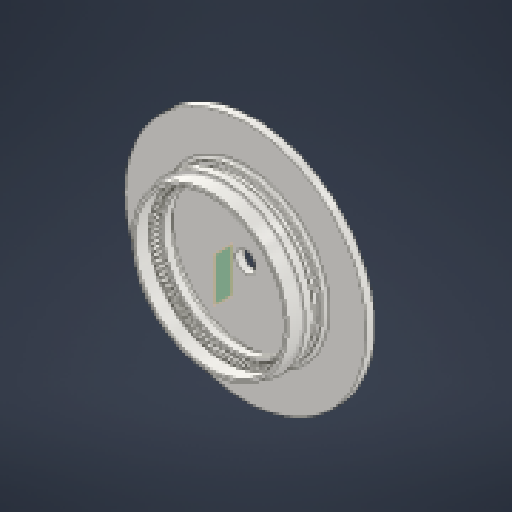
# Autodesk Inventor part: 스퍼 기어1
Saved by Autodesk Inventor 2026.1 (Build 301233020, 233B)
## iProperties
CustomPartVersion: 1
Created: 2025-11-12
Part Number: 스퍼 기어1
Material: Steel
Document SubType Name: Modeling
Designer: jaewook
Categories: <?xml version="1.0" encoding="UTF-16"?> <MemberInstance><Categories><FamilyTemplate><FamilyTemplateParameter ValueType="xs:double" Id="1" ObjectReferenceKey="da_z" ObjectType="kUserParameterObject"/><FamilyTemplateParameter ValueType="xs:double" Id="2" ObjectReferenceKey="da_b" ObjectType="kUserParameterObject"/><FamilyTemplateParameter ValueType="xs:double" Id="3" ObjectReferenceKey="da_beta" ObjectType="kUserParameterObject"/><FamilyTemplateParameter ValueType="xs:double" Id="4" ObjectReferenceKey="da_da" ObjectType="kUserParameterObject"/><FamilyTemplateParameter ValueType="xs:double" Id="5" ObjectReferenceKey="da_aw" ObjectType="kUserParameterObject"/><FamilyTemplateParameter ValueType="xs:string" Id="6" ObjectReferenceKey="EAIAABAAAACIAQAAAAAAAIAAAAAAAAAA" ObjectType="83910656" SubObjectId="SurfaceGeometry"/></FamilyTemplate><ParamToTemplateMap><ParamToTemplate CategoryParameter="//CategoryParameter[@InternalName='046C89C9-8512-4d59-83FE-43B91F4F132A']" TemplateParameter="1"/><ParamToTemplate CategoryParameter="//CategoryParameter[@InternalName='2552DF32-E462-4b46-AEBF-C6C7768E72AC']" TemplateParameter="2"/><ParamToTemplate CategoryParameter="//CategoryParameter[@InternalName='C9EE641D-15FC-4fae-A226-E94C4372FDD7']" TemplateParameter="3"/><ParamToTemplate><ParamToTemplate CategoryParameter="//CategoryParameter[@InternalName='00B6519A-459B-49c7-AD84-2E56D39A5744']" ConstantValue="0.000000"/></ParamToTemplate><ParamToTemplate><ParamToTemplate CategoryParameter="//CategoryParameter[@InternalName='04B31F0E-C7A6-4894-AA32-9629BEFACF47']" ConstantValue="0.950000"/></ParamToTemplate><ParamToTemplate><ParamToTemplate CategoryParameter="//CategoryParameter[@InternalName='43CBEC2E-7847-49e7-A936-2F7889FCB2D9']" ConstantValue="0.250000"/></ParamToTemplate><ParamToTemplate><ParamToTemplate CategoryParameter="//CategoryParameter[@InternalName='B1EFC894-105D-4ebd-86BF-FA20ED196853']" ConstantValue="0.379900"/></ParamToTemplate><ParamToTemplate><ParamToTemplate CategoryParameter="//CategoryParameter[@InternalName='51175063-3D10-4879-93E8-6246FE8B403D']" ConstantValue="2060000000.000000"/></ParamToTemplate><ParamToTemplate><ParamToTemplate CategoryParameter="//CategoryParameter[@InternalName='A3A52E27-4454-46a9-B0BD-C932399B70AF']" ConstantValue="0.300000"/></ParamToTemplate><ParamToTemplate><ParamToTemplate CategoryParameter="//CategoryParameter[@InternalName='91B76062-C214-41d9-B1B9-14D2AB99603D']" ConstantValue="0.200000"/></ParamToTemplate><ParamToTemplate><ParamToTemplate CategoryParameter="//CategoryParameter[@InternalName='374E806E-8B8A-4dda-A9AA-1039D6500AD2']" ConstantValue="5.000000"/></ParamToTemplate><ParamToTemplate><ParamToTemplate CategoryParameter="//CategoryParameter[@InternalName='2D373A89-B862-43d6-8D0B-0CBF12AB9F6C']" ConstantValue="0.349066"/></ParamToTemplate><ParamToTemplate CategoryParameter="//CategoryParameter[@InternalName='37777632-D6A2-4fac-9D53-DB8ACD95C989']" TemplateParameter="4"/><ParamToTemplate CategoryParameter="//CategoryParameter[@InternalName='FD1017F1-B727-4f7e-9707-0F86F1FF9423']" TemplateParameter="5"/><ParamToTemplate><ParamToTemplate CategoryParameter="//CategoryParameter[@InternalName='9E1B4470-B2D3-4ff1-B813-535BB4CDF51A']" ConstantValue="3520000.000000"/></ParamToTemplate><ParamToTemplate><ParamToTemplate CategoryParameter="//CategoryParameter[@InternalName='F8452263-BFF6-458c-9FB1-07C4B99E95CD']" ConstantValue="11400000.000000"/></ParamToTemplate><ParamToTemplate><ParamToTemplate CategoryParameter="//CategoryParameter[@InternalName='3E3BB259-FD49-497f-8171-6EBC954A3479']" ConstantValue="2.000000"/></ParamToTemplate><ParamToTemplate CategoryParameter="//CategoryParameter[@InternalName='27C3BAF2-7550-4e4b-AE2C-0DB134B7D9B7']" TemplateParameter="6"/></ParamToTemplateMap><Category DisplayName="Gear" InternalName="DC85795E-93AB-48d5-8EEE-5A27447B64BD" Mnemonic="Gear"><CategoryParameter DisplayName="z" InternalName="046C89C9-8512-4d59-83FE-43B91F4F132A" Mnemonic="z"/><CategoryParameter DisplayName="b" InternalName="2552DF32-E462-4b46-AEBF-C6C7768E72AC" Mnemonic="b"/><CategoryParameter DisplayName="||b|" InternalName="C9EE641D-15FC-4fae-A226-E94C4372FDD7" Mnemonic="beta"/><CategoryParameter DisplayName="x" InternalName="00B6519A-459B-49c7-AD84-2E56D39A5744" Mnemonic="x"/><CategoryParameter DisplayName="a*" InternalName="04B31F0E-C7A6-4894-AA32-9629BEFACF47" Mnemonic="a"/><CategoryParameter DisplayName="c*" InternalName="43CBEC2E-7847-49e7-A936-2F7889FCB2D9" Mnemonic="c"/><CategoryParameter DisplayName="r|.f|*" InternalName="B1EFC894-105D-4ebd-86BF-FA20ED196853" Mnemonic="rf"/><CategoryParameter DisplayName="E" InternalName="51175063-3D10-4879-93E8-6246FE8B403D" Mnemonic="E"/><CategoryParameter DisplayName="||m|" InternalName="A3A52E27-4454-46a9-B0BD-C932399B70AF" Mnemonic="mi"/><Category DisplayName="SpurGear" InternalName="26C5A22E-A91E-4dfd-A3B3-23CCAFAE1764" Mnemonic="SpurGear"><CategoryParameter DisplayName="m" InternalName="91B76062-C214-41d9-B1B9-14D2AB99603D" Mnemonic="m"/><CategoryParameter DisplayName="P" InternalName="374E806E-8B8A-4dda-A9AA-1039D6500AD2" Mnemonic="PP"/><CategoryParameter DisplayName="||a|" InternalName="2D373A89-B862-43d6-8D0B-0CBF12AB9F6C" Mnemonic="alpha"/><CategoryParameter DisplayName="d|.a|" InternalName="37777632-D6A2-4fac-9D53-DB8ACD95C989" Mnemonic="da"/><CategoryParameter DisplayName="a|.w|" InternalName="FD1017F1-B727-4f7e-9707-0F86F1FF9423" Mnemonic="aw"/><CategoryParameter DisplayName="||s||.Flim|" InternalName="9E1B4470-B2D3-4ff1-B813-535BB4CDF51A" Mnemonic="sFlim"/><CategoryParameter DisplayName="||s||.Hlim|" InternalName="F8452263-BFF6-458c-9FB1-07C4B99E95CD" Mnemonic="sHlim"/><CategoryParameter DisplayName="유형" InternalName="3E3BB259-FD49-497f-8171-6EBC954A3479" Mnemonic="type"/><Category DisplayName="InternalSpurGear" InternalName="7CF704F6-14A9-42f8-93CE-E71DF57C2B55" Mnemonic="InternalSpurGear"><CategoryParameter DisplayName="PitchDiameter" InternalName="27C3BAF2-7550-4e4b-AE2C-0DB134B7D9B7" Mnemonic="IDS_PITCHDIAM"/></Category></Category></Category></Categories></MemberInstance>
Density: 1 g/cm^3
Appearance: Steel
d16: 70.000 mm
d17: 0.000 mm
d45: 0.000 mm
d47: 70.000 mm
d50: 0.000 mm
d51: 0.000 mm
d52: 70.000 mm
Author: jaewook
Autodesk Inventor part; units mm, degrees
sketch "Sketch1" plane through (0, 0, 0) normal (0, 0, 1) x (1, 0, 0)
  circle A0 centre (0, 0) radius 97.02
  dimension "d0" = 194.04
  constraints: 1 centre point
  measures "d0" diameter of A0
extrude "Extrusion1" add sketch "Sketch1" along normal blind 10
ref_plane "Work Plane2" through (0, 0, 5) normal (0, 0, 1) x (1, 0, 0)
sketch "Sketch2" plane through (0, 0, 0) normal (0, 0, -1) x (-1, 0, 0)
  circle A0 centre (0, 0) radius 97.02 projected
  circle A1 centre (0, 0) radius 90
  dimension "d3" = 180
  constraints: 1 centre point, 1 coincident
  measures "d3" diameter of A1
surface extrude "피치 지름" sketch "Sketch2" against normal through all shown no curves A1
ref_plane "Work Plane8" through (0, 0, 0) normal (0.9993908, 0.0348995, 0) x (0, 0, 1)
ref_plane "Work Plane9" through (0, 0, 0) normal (1, 0, 0) x (0, 1, 0)
spur gear teeth "스퍼 기어" teeth 90 pitch diameter 180 tip diameter 176.2 root diameter 184.8 face width 10 start plane through (0, 0, 0) normal (0, 0, -1) x (-1, 0, 0)
sketch "스케치14" plane through (0, 0, 10) normal (0, 0, 1) x (1, 0, 0)
  circle A0 centre (0, 0) radius 97.02 projected
  circle A1 centre (0, 0) radius 93.02
  dimension "d81" = 4
  constraints: 1 centre point, 1 coincident
  measures "d81" radial gap between concentric circles of A1 A0
extrude "돌출9" add sketch "스케치14" along normal blind 17
sketch "스케치15" plane through (0, 0, 0) normal (0, 0, -1) x (-1, 0, 0)
  circle A0 centre (0, 0) radius 97.02 projected
  circle A1 centre (0, 0) radius 92.4
  circle A2 centre (0, 0) radius 95.02
  circle A3 centre (0, 0) radius 85
  dimension "d84" = 184.8
  dimension "d85" = 190.04
  dimension "d86" = 170
  constraints: 3 centre point, 3 coincident
  measures "d84" diameter of A1
  measures "d85" diameter of A2
  measures "d86" diameter of A3
extrude "돌출10" add sketch "스케치15" along normal blind 10 contours A1 | A2
sketch "스케치16" plane through (0, 0, -10) normal (0, 0, -1) x (-1, 0, 0)
  circle A0 centre (0, 0) radius 95.02 projected
  circle A1 centre (0, 0) radius 85 projected
  circle A2 centre (0, 0) radius 90.78
  dimension "d89" = 4.24
  constraints: 1 centre point, 1 coincident
  measures "d89" radial gap between concentric circles of A2 A0
extrude "돌출11" add sketch "스케치16" along normal blind 1 contours A0
sketch "스케치17" plane through (0, 0, -11) normal (0, 0, -1) x (-1, 0, 0)
  circle A0 centre (0, 0) radius 90.78 projected
  circle A1 centre (0, 0) radius 85 projected
  circle A2 centre (0, 0) radius 100.02
  circle A3 centre (0, 0) radius 95.02 projected
  dimension "d150" = 5
  constraints: 1 centre point, 1 coincident
  measures "d150" radial gap between concentric circles of A2 A3
extrude "돌출12" add sketch "스케치17" along normal blind 6.5 contours A2 | A3
sketch "스케치18" plane through (0, 0, -17.5) normal (0, 0, -1) x (-1, 0, 0)
  circle A0 centre (0, 0) radius 90.78 projected
  circle A1 centre (0, 0) radius 150
  circle A2 centre (0, 0) radius 12.5
  dimension "d94" = 300
  dimension "d95" = 25
  constraints: 2 centre point, 2 coincident
  measures "d94" diameter of A1
  measures "d95" diameter of A2
extrude "돌출13" add sketch "스케치18" along normal blind 10 contours A0 | A1
fillet "모깎기2" radius 4 1 edges at (100.02, 0, -17.5)
sketch "스케치4" plane through (0, 0, 0) normal (0, 0, -1) x (-1, 0, 0)
  arc A0 (-13.6576, -91.3851) -> (-12.0606, -91.6095) centre (0, 0) ccw projected
  arc A1 (-19.999, -90.2098) -> (-18.4216, -90.545) centre (0, 0) ccw projected
  arc A2 (-26.243, -88.5949) -> (-24.6928, -89.0395) centre (0, 0) ccw projected
  arc A3 (-32.3592, -86.5485) -> (-30.8438, -87.1001) centre (0, 0) ccw projected
  arc A4 (-38.3177, -84.0804) -> (-36.8444, -84.7364) centre (0, 0) ccw projected
  arc A5 (-44.0895, -81.2027) -> (-42.6656, -81.9598) centre (0, 0) ccw projected
  arc A6 (-49.6465, -77.9294) -> (-48.2789, -78.784) centre (0, 0) ccw projected
  arc A7 (-54.9616, -74.2764) -> (-53.657, -75.2243) centre (0, 0) ccw projected
  arc A8 (-60.009, -70.2615) -> (-58.7736, -71.2981) centre (0, 0) ccw projected
  arc A9 (-64.764, -65.9043) -> (-63.604, -67.0246) centre (0, 0) ccw projected
  arc A10 (-69.2035, -61.2261) -> (-68.1244, -62.4245) centre (0, 0) ccw projected
  arc A11 (-73.3058, -56.2496) -> (-72.313, -57.5204) centre (0, 0) ccw projected
  arc A12 (-77.051, -50.999) -> (-76.1493, -52.3359) centre (0, 0) ccw projected
  arc A13 (-80.4209, -45.4999) -> (-79.6145, -46.8965) centre (0, 0) ccw projected
  arc A14 (-83.3989, -39.7792) -> (-82.6919, -41.2287) centre (0, 0) ccw projected
  arc A15 (-85.9706, -33.8647) -> (-85.3665, -35.3599) centre (0, 0) ccw projected
  arc A16 (-88.1234, -27.7852) -> (-87.6251, -29.319) centre (0, 0) ccw projected
  arc A17 (-89.847, -21.5704) -> (-89.4568, -23.1351) centre (0, 0) ccw projected
  arc A18 (-91.1328, -15.2504) -> (-90.8528, -16.8386) centre (0, 0) ccw projected
  arc A19 (-91.9746, -8.8561) -> (-91.806, -10.46) centre (0, 0) ccw projected
  arc A20 (-92.3683, -2.4188) -> (-92.3121, -4.0304) centre (0, 0) ccw projected
  arc A21 (-92.3121, 4.0304) -> (-92.3683, 2.4188) centre (0, 0) ccw projected
  arc A22 (-91.806, 10.46) -> (-91.9746, 8.8561) centre (0, 0) ccw projected
  arc A23 (-90.8528, 16.8386) -> (-91.1328, 15.2504) centre (0, 0) ccw projected
  arc A24 (-89.4568, 23.1351) -> (-89.847, 21.5704) centre (0, 0) ccw projected
  arc A25 (-87.6251, 29.319) -> (-88.1234, 27.7852) centre (0, 0) ccw projected
  arc A26 (-85.3665, 35.3599) -> (-85.9706, 33.8647) centre (0, 0) ccw projected
  arc A27 (-82.6919, 41.2287) -> (-83.3989, 39.7792) centre (0, 0) ccw projected
  arc A28 (-79.6145, 46.8965) -> (-80.4209, 45.4999) centre (0, 0) ccw projected
  arc A29 (-76.1493, 52.3359) -> (-77.051, 50.999) centre (0, 0) ccw projected
  arc A30 (-72.313, 57.5204) -> (-73.3058, 56.2496) centre (0, 0) ccw projected
  arc A31 (-68.1244, 62.4245) -> (-69.2035, 61.2261) centre (0, 0) ccw projected
  arc A32 (-63.604, 67.0246) -> (-64.764, 65.9043) centre (0, 0) ccw projected
  arc A33 (-58.7736, 71.2981) -> (-60.009, 70.2615) centre (0, 0) ccw projected
  arc A34 (-53.657, 75.2243) -> (-54.9616, 74.2764) centre (0, 0) ccw projected
  arc A35 (-48.2789, 78.784) -> (-49.6465, 77.9294) centre (0, 0) ccw projected
  arc A36 (-42.6656, 81.9598) -> (-44.0895, 81.2027) centre (0, 0) ccw projected
  arc A37 (-36.8444, 84.7364) -> (-38.3177, 84.0804) centre (0, 0) ccw projected
  arc A38 (-30.8438, 87.1001) -> (-32.3592, 86.5485) centre (0, 0) ccw projected
  arc A39 (-24.6928, 89.0395) -> (-26.243, 88.5949) centre (0, 0) ccw projected
  arc A40 (-18.4216, 90.545) -> (-19.999, 90.2098) centre (0, 0) ccw projected
  arc A41 (-12.0606, 91.6095) -> (-13.6576, 91.3851) centre (0, 0) ccw projected
  arc A42 (-5.6409, 92.2277) -> (-7.2496, 92.1152) centre (0, 0) ccw projected
  arc A43 (0.8063, 92.3965) -> (-0.8063, 92.3965) centre (0, 0) ccw projected
  arc A44 (7.2496, 92.1152) -> (5.6409, 92.2277) centre (0, 0) ccw projected
  arc A45 (13.6576, 91.3851) -> (12.0606, 91.6095) centre (0, 0) ccw projected
  arc A46 (19.999, 90.2098) -> (18.4216, 90.545) centre (0, 0) ccw projected
  arc A47 (26.243, 88.5949) -> (24.6928, 89.0395) centre (0, 0) ccw projected
  arc A48 (32.3592, 86.5485) -> (30.8438, 87.1001) centre (0, 0) ccw projected
  arc A49 (38.3177, 84.0804) -> (36.8444, 84.7364) centre (0, 0) ccw projected
  arc A50 (44.0895, 81.2027) -> (42.6656, 81.9598) centre (0, 0) ccw projected
  arc A51 (49.6465, 77.9294) -> (48.2789, 78.784) centre (0, 0) ccw projected
  arc A52 (54.9616, 74.2764) -> (53.657, 75.2243) centre (0, 0) ccw projected
  arc A53 (60.009, 70.2615) -> (58.7736, 71.2981) centre (0, 0) ccw projected
  arc A54 (64.764, 65.9043) -> (63.604, 67.0246) centre (0, 0) ccw projected
  arc A55 (69.2035, 61.2261) -> (68.1244, 62.4245) centre (0, 0) ccw projected
  arc A56 (73.3058, 56.2496) -> (72.313, 57.5204) centre (0, 0) ccw projected
  arc A57 (77.051, 50.999) -> (76.1493, 52.3359) centre (0, 0) ccw projected
  arc A58 (80.4209, 45.4999) -> (79.6145, 46.8965) centre (0, 0) ccw projected
  arc A59 (83.3989, 39.7792) -> (82.6919, 41.2287) centre (0, 0) ccw projected
  arc A60 (85.9706, 33.8647) -> (85.3665, 35.3599) centre (0, 0) ccw projected
  arc A61 (88.1234, 27.7852) -> (87.6251, 29.319) centre (0, 0) ccw projected
  arc A62 (89.847, 21.5704) -> (89.4568, 23.1351) centre (0, 0) ccw projected
  arc A63 (91.1328, 15.2504) -> (90.8528, 16.8386) centre (0, 0) ccw projected
  arc A64 (91.9746, 8.8561) -> (91.806, 10.46) centre (0, 0) ccw projected
  arc A65 (92.3683, 2.4188) -> (92.3121, 4.0304) centre (0, 0) ccw projected
  arc A66 (92.3121, -4.0304) -> (92.3683, -2.4188) centre (0, 0) ccw projected
  arc A67 (91.806, -10.46) -> (91.9746, -8.8561) centre (0, 0) ccw projected
  arc A68 (90.8528, -16.8386) -> (91.1328, -15.2504) centre (0, 0) ccw projected
  arc A69 (89.4568, -23.1351) -> (89.847, -21.5704) centre (0, 0) ccw projected
  arc A70 (87.6251, -29.319) -> (88.1234, -27.7852) centre (0, 0) ccw projected
  arc A71 (85.3665, -35.3599) -> (85.9706, -33.8647) centre (0, 0) ccw projected
  arc A72 (82.6919, -41.2287) -> (83.3989, -39.7792) centre (0, 0) ccw projected
  arc A73 (79.6145, -46.8965) -> (80.4209, -45.4999) centre (0, 0) ccw projected
  arc A74 (76.1493, -52.3359) -> (77.051, -50.999) centre (0, 0) ccw projected
  arc A75 (72.313, -57.5204) -> (73.3058, -56.2496) centre (0, 0) ccw projected
  arc A76 (68.1244, -62.4245) -> (69.2035, -61.2261) centre (0, 0) ccw projected
  arc A77 (63.604, -67.0246) -> (64.764, -65.9043) centre (0, 0) ccw projected
  arc A78 (58.7736, -71.2981) -> (60.009, -70.2615) centre (0, 0) ccw projected
  arc A79 (53.657, -75.2243) -> (54.9616, -74.2764) centre (0, 0) ccw projected
  arc A80 (48.2789, -78.784) -> (49.6465, -77.9294) centre (0, 0) ccw projected
  arc A81 (42.6656, -81.9598) -> (44.0895, -81.2027) centre (0, 0) ccw projected
  arc A82 (36.8444, -84.7364) -> (38.3177, -84.0804) centre (0, 0) ccw projected
  arc A83 (30.8438, -87.1001) -> (32.3592, -86.5485) centre (0, 0) ccw projected
  arc A84 (24.6928, -89.0395) -> (26.243, -88.5949) centre (0, 0) ccw projected
  arc A85 (18.4216, -90.545) -> (19.999, -90.2098) centre (0, 0) ccw projected
  arc A86 (12.0606, -91.6095) -> (13.6576, -91.3851) centre (0, 0) ccw projected
  arc A87 (5.6409, -92.2277) -> (7.2496, -92.1152) centre (0, 0) ccw projected
  arc A88 (-0.8063, -92.3965) -> (0.8063, -92.3965) centre (0, 0) ccw projected
  arc A89 (-7.2496, -92.1152) -> (-5.6409, -92.2277) centre (0, 0) ccw projected
  circle A90 centre (0, 0) radius 97.02 projected
  circle A91 centre (0, 0) radius 92.4
  point P0 (-92.3683, 2.4188)
  point P1 (-92.3121, 4.0304)
  point P2 (-91.9746, 8.8561)
  point P3 (-91.1328, 15.2504)
  point P4 (-89.847, 21.5704)
  point P5 (-88.1234, 27.7852)
  point P6 (-83.3989, 39.7792)
  point P7 (-80.4209, 45.4999)
  point P8 (-79.6145, 46.8965)
  point P9 (-76.1493, 52.3359)
  point P10 (-72.313, 57.5204)
  point P11 (-60.009, 70.2615)
  point P12 (-58.7736, 71.2981)
  point P13 (-54.9616, 74.2764)
  point P14 (-53.657, 75.2243)
  point P15 (-44.0895, 81.2027)
  point P16 (-38.3177, 84.0804)
  point P17 (-32.3592, 86.5485)
  point P18 (-26.243, 88.5949)
  point P19 (-24.6928, 89.0395)
  point P20 (-19.999, 90.2098)
  point P21 (-18.4216, 90.545)
  point P22 (-13.6576, 91.3851)
  point P23 (-12.0606, 91.6095)
  point P24 (-7.2496, 92.1152)
  point P25 (-0.8063, 92.3965)
  point P26 (0.8063, 92.3965)
  point P27 (5.6409, 92.2277)
  point P28 (7.2496, 92.1152)
  point P29 (12.0606, 91.6095)
  point P30 (18.4216, 90.545)
  point P31 (24.6928, 89.0395)
  point P32 (30.8438, 87.1001)
  point P33 (36.8444, 84.7364)
  point P34 (38.3177, 84.0804)
  point P35 (42.6656, 81.9598)
  point P36 (48.2789, 78.784)
  point P37 (49.6465, 77.9294)
  point P38 (54.9616, 74.2764)
  point P39 (58.7736, 71.2981)
  point P40 (63.604, 67.0246)
  point P41 (68.1244, 62.4245)
  point P42 (72.313, 57.5204)
  point P43 (73.3058, 56.2496)
  point P44 (79.6145, 46.8965)
  point P45 (80.4209, 45.4999)
  point P46 (85.3665, 35.3599)
  point P47 (87.6251, 29.319)
  point P48 (89.4568, 23.1351)
  point P49 (89.847, 21.5704)
  point P50 (90.8528, 16.8386)
  point P51 (91.1328, 15.2504)
  point P52 (91.806, 10.46)
  point P53 (91.9746, 8.8561)
  point P54 (92.3683, -2.4188)
  point P55 (92.3121, -4.0304)
  point P56 (91.9746, -8.8561)
  point P57 (91.1328, -15.2504)
  point P58 (89.847, -21.5704)
  point P59 (88.1234, -27.7852)
  point P60 (85.9706, -33.8647)
  point P61 (72.313, -57.5204)
  point P62 (60.009, -70.2615)
  point P63 (58.7736, -71.2981)
  point P64 (54.9616, -74.2764)
  point P65 (53.657, -75.2243)
  point P66 (49.6465, -77.9294)
  point P67 (44.0895, -81.2027)
  point P68 (38.3177, -84.0804)
  point P69 (32.3592, -86.5485)
  point P70 (26.243, -88.5949)
  point P71 (19.999, -90.2098)
  point P72 (18.4216, -90.545)
  point P73 (13.6576, -91.3851)
  point P74 (12.0606, -91.6095)
  point P75 (7.2496, -92.1152)
  point P76 (0.8063, -92.3965)
  point P77 (-0.8063, -92.3965)
  point P78 (-7.2496, -92.1152)
  point P79 (-12.0606, -91.6095)
  point P80 (-18.4216, -90.545)
  point P81 (-24.6928, -89.0395)
  point P82 (-26.243, -88.5949)
  point P83 (-30.8438, -87.1001)
  point P84 (-32.3592, -86.5485)
  point P85 (-36.8444, -84.7364)
  point P86 (-38.3177, -84.0804)
  point P87 (-48.2789, -78.784)
  point P88 (-53.657, -75.2243)
  point P89 (-58.7736, -71.2981)
  point P90 (-63.604, -67.0246)
  point P91 (-64.764, -65.9043)
  point P92 (-69.2035, -61.2261)
  point P93 (-72.313, -57.5204)
  point P94 (-73.3058, -56.2496)
  point P95 (-76.1493, -52.3359)
  point P96 (-77.051, -50.999)
  point P97 (-82.6919, -41.2287)
  point P98 (-83.3989, -39.7792)
  point P99 (-85.3665, -35.3599)
  point P100 (-87.6251, -29.319)
  point P101 (-90.8528, -16.8386)
  point P102 (-91.806, -10.46)
  point P103 (-92.3121, -4.0304)
  constraints: 1 coincident, 1 other
sketch "스케치6" plane through (0, 0, -10) normal (0, 0, -1) x (-1, 0, 0)
  arc A0 (51.6266, -76.6319) -> (92.1785, -6.394) centre (0, 0) ccw projected
  circle A1 centre (0, 0) radius 101.64 projected
  arc A2 (92.1785, 6.394) -> (51.6266, 76.6319) centre (0, 0) ccw projected
  circle A3 centre (0, 0) radius 97.02
  dimension "d69" = 4.62
  constraints: 1 centre point, 1 coincident
  measures "d69" radial gap between concentric circles of A0 A3
sketch "스케치7" plane through (0, 0, -10) normal (0, 0, -1) x (-1, 0, 0)
  circle A0 centre (0, 0) radius 97.02 projected
  arc A1 (51.6266, -76.6319) -> (92.1785, -6.394) centre (0, 0) ccw projected
  arc A2 (-40.5519, -83.0259) -> (40.5519, -83.0259) centre (0, 0) ccw projected
  arc A3 (-92.1785, -6.394) -> (-51.6266, -76.6319) centre (0, 0) ccw projected
  arc A4 (-51.6266, 76.6319) -> (-92.1785, 6.394) centre (0, 0) ccw projected
  arc A5 (40.5519, 83.0259) -> (-40.5519, 83.0259) centre (0, 0) ccw projected
  arc A6 (92.1785, 6.394) -> (51.6266, 76.6319) centre (0, 0) ccw projected
  circle A7 centre (0, 0) radius 97.02
  circle A8 centre (0, 0) radius 92.4
  point P0 (-92.1785, -6.394)
  point P1 (-92.1785, 6.394)
  point P2 (-51.6266, 76.6319)
  point P3 (-40.5519, 83.0259)
  point P4 (40.5519, 83.0259)
  point P5 (92.1785, 6.394)
  point P6 (40.5519, -83.0259)
  point P7 (-40.5519, -83.0259)
  point P8 (-51.6266, -76.6319)
  constraints: 2 centre point, 2 coincident, 2 concentric
sketch "스케치8" plane through (0, 0, -14) normal (0, 0, -1) x (-1, 0, 0)
  circle A0 centre (0, 0) radius 97.02 projected
  circle A1 centre (0, 0) radius 92.4 projected
  circle A2 centre (0, 0) radius 102.45
  constraints: 1 centre point, 1 coincident
sketch "스케치9" plane through (0, 0, -14) normal (0, 0, 1) x (1, 0, 0)
  circle A0 centre (0, 0) radius 102.45 projected
  circle A1 centre (0, 0) radius 97.02 projected
sketch "스케치10" plane through (0, 0, -18) normal (0, 0, -1) x (-1, 0, 0)
  circle A0 centre (0, 0) radius 102.45 projected
  circle A1 centre (0, 0) radius 92.4 projected
  circle A2 centre (0, 0) radius 150
  dimension "d78" = 300
  constraints: 1 centre point, 1 coincident
  measures "d78" diameter of A2
mirror "미러1" about plane through (0, 0, 0) normal (1, 0, 0)
sketch "스케치25" plane through (0, 0, -27.5) normal (0, 0, -1) x (-1, 0, 0)
  circle A0 centre (0, 0) radius 150 projected
  circle A1 centre (0, 0) radius 12.5 projected
  line L0 (63.5, -15) -> (69.5, -15)
  line L1 (69.5, -15) -> (69.5, 15)
  line L2 (69.5, 15) -> (63.5, 15)
  line L3 (63.5, 15) -> (63.5, -15)
  line L4 (0, 0) -> (150, 0) construction
  line L5 (0, 0) -> (0, 150) construction
  line L6 (-63.5, -15) -> (-69.5, -15)
  line L7 (-69.5, -15) -> (-69.5, 15)
  line L8 (-69.5, 15) -> (-63.5, 15)
  line L9 (-63.5, 15) -> (-63.5, -15)
  dimension "d139" = 63.5
  dimension "d140" = 6
  dimension "d141" = 30
  constraints: 20 end point, 4 symmetric about line, 2 parallel, 2 point on circle, 1 horizontal, 1 perpendicular, 1 vertical, 1 other
  measures "d139" distance from line of L3 A0.centre
  measures "d140" distance of L1.end L2.end
  measures "d141" distance of L0.end L1.end
extrude "돌출19" add sketch "스케치25" along normal blind 60 contours L3 L2 L1 L0 | L6 L7 L8 L9
sketch "스케치26" plane through (-69.5, -15, -27.5) normal (-1, 0, 0) x (0, 0, 1)
  line L0 (0, 30) -> (0, 0) projected
  line L1 (-60, 0) -> (-60, 30) projected
  circle A0 centre (-50, 15) radius 2
  point P0 (27.5, 15)
  point P1 (-60, 15)
  dimension "d144" = 4
  dimension "d145" = 50
  constraints: 1 centre point, 1 horizontal alignment, 1 midpoint
  measures "d144" diameter of A0
  measures "d145" distance from line of A0.centre L0
extrude "돌출20" cut sketch "스케치26" against normal through all
sketch "스케치29" plane through (0, 0, 0) normal (1, 0, 0) x (0, 1, 0)
  line L0 (-100.02, -11) -> (100.02, -11) projected
  line L1 (101.32, 0) -> (95.02, -6.3)
  line L2 (-97.02, 0) -> (97.02, 0) projected
  line L3 (95.02, 0) -> (95.02, -11) projected
  line L4 (95.02, 0) -> (95.02, -11) projected
  line L5 (0, -11) -> (0, 0)
  line L6 (101.32, 0) -> (97.02, 0)
  point P0 (97.3, -4.02)
  point P1 (97.3, -4.02)
  dimension "d153" = 6.98
  dimension "d154" = 45
  dimension "d155" = 194.6
  constraints: 6 end point, 2 point on line, 1 coincident, 1 horizontal, 1 midpoint, 1 perpendicular
  measures "d153" distance from line of point (97.3, -4.02) L0
  measures "d154" angle of L2 L1
  measures "d155" diameter of point (97.3, -4.02) L5
revolve "회전2" add sketch "스케치29" angle 360 about axis through (0, 0, -11) along (0, 0, 1) separate body contours L3 L2 L6 L1
sketch "스케치30" plane through (0, 0, 0) normal (0, 0, 1) x (1, 0, 0)
  circle A0 centre (0, 0) radius 95.02 projected
  circle A1 centre (0, 0) radius 101.32 projected
  dimension "d56" = 238.049
  dimension "d57" = 255.5606
  dimension "d60" = 360
  dimension "d64" = 360
extrude "돌출22" add sketch "스케치30" along normal blind 22 bodies 2
ref_plane "작업 평면12" through (0, 0, 0) normal (1, 0, 0) x (0, 1, 0)
equation "\"d1\" = da_b"
equation "\"d3\" = da_d"
equation "\"d16\" = da_aw"
equation "\"d47\" = da_aw"
equation "\"d52\" = da_aw"
equation "\"da_b\" = 10"
equation "\"da_d\" = 180"
equation "\"da_aw\" = 70"
body "Solid1"
body "Srf1"
